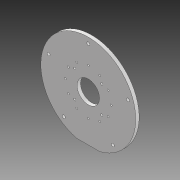
# Autodesk Inventor part: J0_motorbracket
Saved by Autodesk Inventor 2020 (Build 240168000, 168)
## iProperties
Created: 2021-03-20
Part Number: J0_motorbracket
Material: Generic
Document SubType Name: Modeling
Designer: DDeGo
Density: 1 g/cm^3
Appearance: Default
Author: DDeGo
Autodesk Inventor part; units mm, degrees
ref_plane "YZ Plane" through (0, 0, 0) normal (1, 0, 0) x (0, 1, 0)
ref_plane "XZ Plane" through (0, 0, 0) normal (0, 1, 0) x (-1, 0, 0)
ref_plane "XY Plane" through (0, 0, 0) normal (0, 0, 1) x (1, 0, 0)
sketch "Sketch1" plane through (0, 0, 0) normal (0, 0, 1) x (1, 0, 0)
  circle A0 centre (-42.6144, -58.6537) radius 2.6
  circle A1 centre (-68.9516, 22.4037) radius 2.6
  circle A2 centre (42.6144, -58.6537) radius 2.6
  circle A3 centre (0, 72.5) radius 2.6
  circle A4 centre (68.9516, 22.4037) radius 2.6
  arc A5 (82.5, 0) -> (-82.5, 0) centre (0, 0) ccw
  line L0 (-82.5, 0) -> (-82.5, -80)
  line L1 (-82.5, -80) -> (82.5, -80)
  line L2 (82.5, -80) -> (82.5, 0)
  circle A6 centre (0, 0) radius 62.5
  constraints: 7 centre point, 6 end point, 2 point on circle
extrude "Extrusion1" add sketch "Sketch1" along normal blind 6 contours L2 L1 L0 A5 | A6
sketch "Sketch2" plane through (0, 0, 6) normal (0, 0, 1) x (1, 0, 0)
  circle A0 centre (0, 0) radius 19.5
  line L0 (-23.5, -23.5) -> (23.5, -23.5) construction
  line L1 (23.5, -23.5) -> (23.5, 23.5) construction
  line L2 (23.5, 23.5) -> (-23.5, 23.5) construction
  line L3 (-23.5, 23.5) -> (-23.5, -23.5) construction
  line L4 (-23.5, -23.5) -> (23.5, 23.5) construction
  line L5 (23.5, -23.5) -> (-23.5, 23.5) construction
  circle A1 centre (-23.5, 23.5) radius 2
  circle A2 centre (23.5, 23.5) radius 2
  circle A3 centre (23.5, -23.5) radius 2
  circle A4 centre (-23.5, -23.5) radius 2
  dimension "d2" = 39
  dimension "d3" = 47
  dimension "d4" = 4
  constraints: 12 end point, 5 centre point, 5 coincident, 3 equal radius, 2 midpoint, 2 parallel, 2 perpendicular, 1 horizontal
  measures "d2" diameter of A0
  measures "d3" distance of L2.end L0.start
  measures "d4" diameter of A1
extrude "Extrusion2" cut sketch "Sketch2" against normal through all
sketch "Sketch3" plane through (0, 0, 6) normal (0, 0, 1) x (1, 0, 0)
  arc A0 (82.5, 0) -> (-82.5, 0) centre (0, 0) ccw projected
  circle A1 centre (0, 0) radius 82.5
  circle A2 centre (0, 0) radius 147.6285
  constraints: 2 coincident, 1 centre point, 3 other
extrude "Extrusion3" cut sketch "Sketch3" against normal through all
sketch "Sketch4" plane through (0, 0, 6) normal (0, 0, 1) x (1, 0, 0)
  circle A0 centre (0, 0) radius 40 construction
  circle A1 centre (-40, 0) radius 1.6
  line L0 (-40, 0) -> (0, 0) construction
  line L1 (-34.641, -20) -> (0, 0) construction
  circle A2 centre (-34.641, -20) radius 1.6
  line L2 (-20, -34.641) -> (0, 0) construction
  circle A3 centre (-20, -34.641) radius 1.6
  line L3 (0, -40) -> (0, 0) construction
  circle A4 centre (0, -40) radius 1.6
  line L4 (20, -34.641) -> (0, 0) construction
  circle A5 centre (20, -34.641) radius 1.6
  line L5 (34.641, -20) -> (0, 0) construction
  circle A6 centre (34.641, -20) radius 1.6
  line L6 (40, 0) -> (0, 0) construction
  circle A7 centre (40, 0) radius 1.6
  line L7 (34.641, 20) -> (0, 0) construction
  circle A8 centre (34.641, 20) radius 1.6
  line L8 (20, 34.641) -> (0, 0) construction
  circle A9 centre (20, 34.641) radius 1.6
  line L9 (0, 40) -> (0, 0) construction
  circle A10 centre (0, 40) radius 1.6
  line L10 (-20, 34.641) -> (0, 0) construction
  circle A11 centre (-20, 34.641) radius 1.6
  line L11 (-34.641, 20) -> (0, 0) construction
  circle A12 centre (-34.641, 20) radius 1.6
  dimension "d9" = 80
  dimension "d10" = 3.2
  dimension "d13" = 360
  constraints: 24 end point, 12 centre point, 1 coincident, 1 horizontal, 1 horizontal alignment, 51 other
  measures "d10" diameter of A1
extrude "Extrusion4" cut sketch "Sketch4" against normal through all
body "Solid1"
